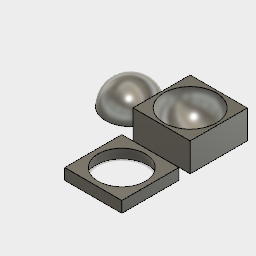
design (Autodesk Fusion 360 design; units mm, degrees)
Autodesk Fusion 360 part; units mm, degrees
sphere "SpherePrimitive1" add diameter 40 placed x (1, 0, 0) y (0, 0, -1) z (0, 1, 0) at (0, 0, 0) makes body 1
delete_face "DeleteFace1" 1 faces at (18.9615, 4.7276, -4.2557) on bodies 1
sphere "SpherePrimitive2" add diameter 42 placed x (1, 0, 0) y (0, 0, -1) z (0, 1, 0) at (0, 0, 0) separate body makes body 2
box "BoxPrimitive1" add length 46 width 46 height 46 placed x (0, 0, -1) y (-1, 0, 0) z (0, 1, 0) at (46, 0, 0) separate body makes body 3
move_body "MoveBody1" bodies 2 to x (1, 0, 0) y (0, 1, 0) z (0, 0, 1) at (0, 23, 0)
move_body "MoveBody2" bodies 2 to x (1, 0, 0) y (0, 1, 0) z (0, 0, 1) at (0, 0, -23)
move_body "MoveBody3" bodies 2 to x (1, 0, 0) y (0, 1, 0) z (0, 0, 1) at (23, 0, 0)
sphere "SpherePrimitive3" add diameter 40 placed x (1, 0, 0) y (0, 1, 0) z (0, 0, 1) at (5, 15, 0) separate body makes body 4
move_body "MoveBody4" bodies 4 to x (1, 0, 0) y (0, 1, 0) z (0, 0, 1) at (0, 5, 0)
move_body "MoveBody5" bodies 4 to x (1, 0, 0) y (0, 1, 0) z (0, 0, 1) at (0, 3, 0)
move_body "MoveBody6" bodies 4 to x (1, 0, 0) y (0, 1, 0) z (0, 0, 1) at (0, 0, -23)
combine "Combine1" operation cut target body 3 tool bodies 2 keep tools
extrude "Extrude1" cut 1 faces at (15.3333, 46, -15.3333) along direction (0, -1, 0) blind 14 on bodies 3 bodies 2 3
move_body "MoveBody8" bodies 4 to x (1, 0, 0) y (0, 1, 0) z (0, 0, 1) at (-30, -2, 0)
move_body "MoveBody9" bodies 4 to x (1, 0, 0) y (0, 1, 0) z (0, 0, 1) at (0, -1, 0)
box "BoxPrimitive3" cut length 99.2987 width 58.0087 height 20 placed x (0, 0, 1) y (1, 0, 0) z (0, 1, 0) at (-58.0087, 0, -79.2987) bodies 4
move_body "MoveBody10" bodies 4 to x (1, 0, 0) y (0, 1, 0) z (0, 0, 1) at (0, -20, 0)
copy_body "CopyPasteBodies1" bodies 3 makes body 5
move_body "MoveBody11" bodies 5 to x (1, 0, 0) y (0, 1, 0) z (0, 0, 1) at (0, 0, 55)
box "BoxPrimitive4" cut length 70.1585 width 78.149 height 23 placed x (0, 0, 1) y (1, 0, 0) z (0, 1, 0) at (-20, 0, 4.8415) bodies 5
copy_body "CopyPasteBodies2" bodies 5 makes body 6
move_body "MoveBody12" bodies 6 to x (1, 0, 0) y (0, 1, 0) z (0, 0, 1) at (0, 0, -55)
combine "Combine2" operation cut target body 3 tool bodies 6
move_body "MoveBody13" bodies 5 to x (1, 0, 0) y (0, 1, 0) z (0, 0, 1) at (0, -23, 0)
delete_body "RemoveBody1" bodies 2
extrude "Extrude2" [rolled back] along distance -23 taper angle 0
move_body "MoveBody7" [rolled back]
boxprimitive "BoxPrimitive2" [rolled back] distance x 65 distance y 80 distance z 20 offset distance x 0 offset distance y 0
hole "Hole1" [rolled back] hole depth 20 hole diameter 20 tip angle 118
